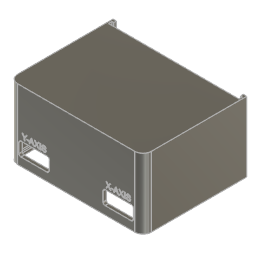
PCB Top Enclosure (Autodesk Fusion 360 design; units mm, degrees)
part number: 2026-07-12-14-24-08-666
Autodesk Fusion 360 part; units mm, degrees
sketch "Sketch1" plane through (0, 0, 0) normal (0, 0, 1) x (1, 0, 0)
  line L0 (-48.5, 1.25) -> (48.5, 1.25)
  line L1 (48.5, 1.25) -> (48.5, -1.25)
  line L2 (48.5, -1.25) -> (-48.5, -1.25)
  line L3 (-48.5, -1.25) -> (-48.5, 1.25)
  line L4 (-48.5, 1.25) -> (48.5, -1.25) construction
  line L5 (48.5, 1.25) -> (-48.5, -1.25) construction
  line L6 (-48.5, 1.25) -> (-46, 1.25)
  line L7 (-46, 1.25) -> (-46, 74.25)
  line L8 (-46, 74.25) -> (-48.5, 74.25)
  line L9 (-48.5, 74.25) -> (-48.5, 1.25)
  line L10 (48.5, 1.25) -> (46, 1.25)
  line L11 (46, 1.25) -> (46, 74.25)
  line L12 (46, 74.25) -> (48.5, 74.25)
  line L13 (48.5, 74.25) -> (48.5, 1.25)
  dimension "d1" = 2.5
  dimension "d2" = 97
  dimension "d3" = 73
  constraint horizontal L0
  constraint perpendicular L0 L1
  constraint parallel L0 L2
  constraint parallel L1 L3
  constraint coincident L4 origin
  constraint coincident L5 origin
  constraint horizontal L6
  constraint vertical L7
  constraint horizontal L8
  constraint vertical L9
  constraint horizontal L10
  constraint vertical L11
  constraint horizontal L12
  constraint vertical L13
  constraint equal L7 L11
  constraint equal L8 L12
  constraint equal L3 L8
  measures "d1" distance of L7.end L8.end
  measures "d2" distance of L1.end L2.end
  measures "d3" distance of L0.end L12.end
extrude "Extrude1" add sketch "Sketch1" along normal blind 50.8
sketch "Sketch2" plane through (0, 0, 50.8) normal (0, 0, 1) x (-1, 0, 0)
  line L0 (46, -1.25) -> (46, -74.25)
  line L1 (46, -74.25) -> (48.5, -74.25)
  line L2 (48.5, -74.25) -> (48.5, 1.25)
  line L3 (48.5, 1.25) -> (-48.5, 1.25)
  line L4 (-48.5, 1.25) -> (-48.5, -74.25)
  line L5 (-48.5, -74.25) -> (-46, -74.25)
  line L6 (-46, -74.25) -> (-46, -1.25)
  line L7 (-46, -1.25) -> (46, -1.25)
  line L8 (-48.5, 1.25) -> (48.5, 1.25)
  line L9 (48.5, 1.25) -> (48.5, -69.5003)
  line L10 (48.5, -69.5003) -> (-48.5, -69.5003)
  line L11 (-48.5, -69.5003) -> (-48.5, 1.25)
  dimension "d35" = 70.7503
  constraint horizontal L8
  constraint vertical L9
  constraint horizontal L10
  constraint vertical L11
  constraint coincident L2 L9.end
  constraint coincident L3.end L4.start
  measures "d35" distance of L2.end L9.end
extrude "Extrude2" add sketch "Sketch2" against normal blind 2 contours L0 L6 L7 L10
sketch "Sketch3" plane through (0, 74.25, 0) normal (0, 1, 0) x (-1, 0, 0)
  line L0 (-48.5, 0) -> (-46, 0)
  line L1 (-46, 0) -> (-46, 50.8)
  line L2 (-46, 50.8) -> (-48.5, 50.8)
  line L3 (-48.5, 50.8) -> (-48.5, 0)
  line L4 (-47.25, 2) -> (47.25, 2)
  line L5 (47.25, 2) -> (47.25, 4.5)
  line L6 (47.25, 4.5) -> (-47.25, 4.5)
  line L7 (-47.25, 4.5) -> (-47.25, 2)
  line L8 (48.5, 0) -> (48.5, 50.8)
  line L9 (46, 0) -> (-46, 0)
  dimension "d12" = 2.5
  dimension "d13" = 2.5
  dimension "d14" = 1.25
  dimension "d15" = 1.25
  dimension "d16" = 2
  constraint horizontal L4
  constraint vertical L5
  constraint horizontal L6
  constraint vertical L7
  measures "d12" distance of L4 L6
  measures "d13" distance of L1.end L2.end
  measures "d14" distance of L3 L7
  measures "d15" distance of L4.end L8
  measures "d16" distance of L4 L9
extrude "Extrude3" cut sketch "Sketch3" against normal blind 74.25 contours L1 L4 L6 L7 | L1 L4 L5 L6
fillet "Fillet6" radius 3 2 edges at (47.25, 0, 3.25) (-47.25, 0, 3.25)
fillet "Fillet7" radius 3 4 edges at (-46, 1.25, 1) (-46, 1.25, 26.65) (46, 1.25, 1) (46, 1.25, 26.65)
fillet "Fillet8" radius 6 2 edges at (-48.5, -1.25, 25.4) (48.5, -1.25, 25.4)
sketch "Sketch4" plane through (0, 74.25, 0) normal (0, 1, 0) x (-1, 0, 0)
  line L0 (-46, 2) -> (-47.25, 2)
  line L1 (-47.25, 2) -> (-47.25, 4.5)
  line L2 (-47.25, 4.5) -> (-46, 4.5)
  line L3 (-46, 4.5) -> (-46, 50.8)
  line L4 (-46, 50.8) -> (-48.5, 50.8)
  line L5 (-48.5, 50.8) -> (-48.5, 0)
  line L6 (-48.5, 0) -> (-46, 0)
  line L7 (-46, 0) -> (-46, 2)
  line L8 (-56.493, 66.6697) -> (57.302, 66.6697)
  line L9 (57.302, 66.6697) -> (57.302, -11.9997)
  line L10 (57.302, -11.9997) -> (-56.493, -11.9997)
  line L11 (-56.493, -11.9997) -> (-56.493, 66.6697)
  constraint horizontal L8
  constraint vertical L9
  constraint horizontal L10
  constraint vertical L11
extrude "Extrude4" cut sketch "Sketch4" against normal blind 0.25 contours L0 L1 L2 L3 L4 L5 L6 L7 | L8 L9 L10 L11
sketch "Sketch5" plane through (0, -1.25, 0) normal (0, -1, 0) x (1, 0, 0)
  line L0 (42.5, 0) -> (42.5, 50.8)
  line L1 (42.5, 50.8) -> (-42.5, 50.8)
  line L2 (-42.5, 50.8) -> (-42.5, 0)
  line L3 (-42.5, 0) -> (42.5, 0)
  line L4 (41.5, 6) -> (19.5, 6)
  line L5 (19.5, 6) -> (19.5, 16)
  line L6 (19.5, 16) -> (41.5, 16)
  line L7 (41.5, 16) -> (41.5, 6)
  line L8 (-19.5, 6) -> (-41.5, 6)
  line L9 (-41.5, 6) -> (-41.5, 16)
  line L10 (-41.5, 16) -> (-19.5, 16)
  line L11 (-19.5, 16) -> (-19.5, 6)
  line L12 (48.5, 0) -> (48.5, 50.8)
  line L13 (-48.5, 50.8) -> (-48.5, 0)
  dimension "d36" = 22
  dimension "d37" = 10
  dimension "d38" = 7
  dimension "d39" = 7
  dimension "d40" = 6
  constraint horizontal L4
  constraint vertical L5
  constraint horizontal L6
  constraint vertical L7
  constraint horizontal L8
  constraint vertical L9
  constraint horizontal L10
  constraint vertical L11
  constraint equal L4 L8
  constraint equal L5 L11
  constraint collinear L4 L8
  measures "d36" distance of L4.start L4.end
  measures "d37" distance of L4.end L5.end
  measures "d38" distance of L7 L12
  measures "d39" distance of L9 L13
  measures "d40" distance of L3 L4
extrude "Extrude5" cut sketch "Sketch5" against normal blind 5 contours L4 L5 L6 L7 | L8 L9 L10 L11
fillet "Fillet9" radius 1.5 8 edges at (-41.5, 0, 16) (-19.5, 0, 16) (-41.5, 0, 6) (-19.5, 0, 6) (41.5, 0, 6) (41.5, 0, 16) (19.5, 0, 16) (19.5, 0, 6)
sketch "Sketch6" plane through (0, 0, 50.8) normal (0, 0, 1) x (-1, 0, 0)
  line L0 (48.5, -74) -> (48.5, -4.75)
  arc A0 (48.5, -4.75) -> (42.5, 1.25) centre (42.5, -4.75) ccw
  line L1 (42.5, 1.25) -> (-42.5, 1.25)
  arc A1 (-42.5, 1.25) -> (-48.5, -4.75) centre (-42.5, -4.75) ccw
  line L2 (-48.5, -4.75) -> (-48.5, -74)
  line L3 (-46, -74) -> (-46, -69.5003)
  line L4 (-46, -69.5003) -> (46, -69.5003)
  line L5 (46, -69.5003) -> (46, -74)
  line L6 (-47.25, -72.0003) -> (47.25, -72.0003)
  line L7 (47.25, -72.0003) -> (47.25, -69.5003)
  line L8 (47.25, -69.5003) -> (-47.25, -69.5003)
  line L9 (-47.25, -69.5003) -> (-47.25, -72.0003)
  line L10 (46, -74) -> (48.5, -74)
  line L11 (-48.5, -74) -> (-46, -74)
  dimension "d45" = 2.5
  dimension "d46" = 2.5
  dimension "d47" = 1.25
  dimension "d48" = 1.25
  constraint horizontal L6
  constraint vertical L7
  constraint horizontal L8
  constraint vertical L9
  constraint collinear L4 L8
  measures "d45" distance of L6.start L8.end
  measures "d46" distance of L2.end L3.start
  measures "d47" distance of L2 L9
  measures "d48" distance of L0 L7
extrude "Extrude6" cut sketch "Sketch6" against normal up to surface (48.8 mm away) contours L5 L6 L7 L8 | L3 L6 L8 L9
sketch "Sketch7" plane through (0, -1.25, 0) normal (0, -1, 0) x (1, 0, 0)
  line L0 (19.5, 7.5) -> (19.5, 14.5)
  arc A0 (21, 16) -> (19.5, 14.5) centre (21, 14.5) ccw
  line L1 (21, 16) -> (40, 16)
  arc A1 (41.5, 14.5) -> (40, 16) centre (40, 14.5) ccw
  line L2 (41.5, 14.5) -> (41.5, 7.5)
  arc A2 (40, 6) -> (41.5, 7.5) centre (40, 7.5) ccw
  line L3 (40, 6) -> (21, 6)
  arc A3 (19.5, 7.5) -> (21, 6) centre (21, 7.5) ccw
  line L4 (-41.5, 7.5) -> (-41.5, 14.5)
  arc A4 (-40, 16) -> (-41.5, 14.5) centre (-40, 14.5) ccw
  line L5 (-40, 16) -> (-21, 16)
  arc A5 (-19.5, 14.5) -> (-21, 16) centre (-21, 14.5) ccw
  line L6 (-19.5, 14.5) -> (-19.5, 7.5)
  arc A6 (-21, 6) -> (-19.5, 7.5) centre (-21, 7.5) ccw
  line L7 (-21, 6) -> (-40, 6)
  arc A7 (-41.5, 7.5) -> (-40, 6) centre (-40, 7.5) ccw
  line L8 (42.5, 0) -> (42.5, 50.8)
  line L9 (42.5, 50.8) -> (-42.5, 50.8)
  line L10 (-42.5, 50.8) -> (-42.5, 0)
  line L11 (-42.5, 0) -> (42.5, 0)
  line L12 (-40.5, 17) -> (-20.5, 17) construction
  line L13 (-20.5, 17) -> (-20.5, 22) construction
  line L14 (-20.5, 22) -> (-40.5, 22) construction
  line L15 (-40.5, 22) -> (-40.5, 17) construction
  line L16 (20.5, 17) -> (40.5, 17) construction
  line L17 (40.5, 17) -> (40.5, 22) construction
  line L18 (40.5, 22) -> (20.5, 22) construction
  line L19 (20.5, 22) -> (20.5, 17) construction
  dimension "d51" = 4
  dimension "d53" = 5
  dimension "d54" = 20
  dimension "d55" = 17
  dimension "d56" = 19
  dimension "d57" = 9.5
  dimension "d58" = 4
  dimension "d60" = 5
  dimension "d61" = 20
  dimension "d62" = 9.5
  dimension "d63" = 17
  text T0 "Y-AXIS" font "Arial" height 4 align centre middle in box 20 x 5 at (-40.5, 17) x (1, 0) y (0, 1) spacing 1 kerned
  text T1 "X-AXIS" font "Arial" height 4 align centre middle in box 20 x 5 at (20.5, 17) x (1, 0) y (0, 1) spacing 1 kerned
  constraint horizontal L14
  constraint horizontal L18
  measures "d55" distance of L11 L12
  measures "d56" distance of A4.start L5.end
  measures "d57" distance of A4.start
  measures "d62" distance of L1.end
  measures "d63" distance of L11 L16
extrude "Extrude7" cut sketch "Sketch7" against normal blind 1 text T1 T0
equation "d14 = d13 / 2"
equation "d15 = d14"
equation "d17 = -72.5 mm - 1.75 mm"
equation "d33 = -4.75 mm + 2.5 mm + 2 mm"
equation "d35 = 68.9813377182 mm + 1.769 mm"
equation "d40 = 2.5 mm + 2 mm + 1.5 mm"
equation "d47 = d46 / 2"
equation "d48 = d46 / 2"
equation "d52 = 'Y-AXIS'"
equation "d57 = d56 / 2"
equation "d59 = 'X-AXIS'"
equation "d62 = d57"
equation "d63 = d55"
